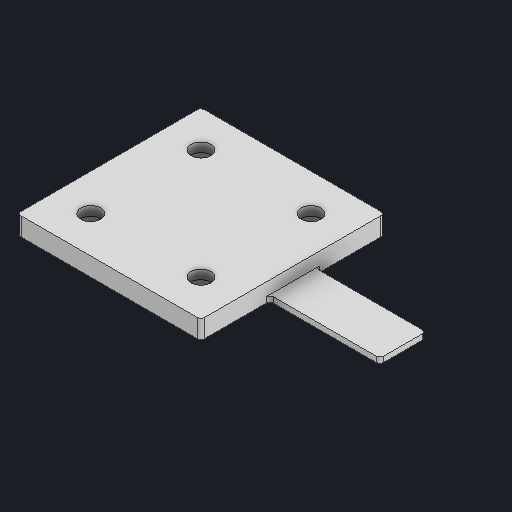
# Autodesk Inventor part: cradle_base
Saved by Autodesk Inventor 2025 (Build 290162010, 162A)
## iProperties
Created: 2024-06-21
Part Number: cradle_base
Material: Generic
Document SubType Name: Modeling
Designer: mihir
Density: 1 g/cm^3
Appearance: Default
Author: mihir
Autodesk Inventor part; units mm, degrees
ref_plane "YZ Plane" through (0, 0, 0) normal (1, 0, 0) x (0, 1, 0)
ref_plane "XZ Plane" through (0, 0, 0) normal (0, 1, 0) x (-1, 0, 0)
ref_plane "XY Plane" through (0, 0, 0) normal (0, 0, 1) x (1, 0, 0)
sketch "Sketch1" plane through (0, 0, 0) normal (0, 1, 0) x (-1, 0, 0)
  line L0 (100, 0) -> (0, 0)
  line L1 (0, 0) -> (0, -100)
  line L2 (0, -100) -> (100, -100)
  line L3 (100, -100) -> (100, 0)
  dimension "d0" = 100
  constraints: 8 end point, 2 parallel, 2 perpendicular, 1 coincident, 1 horizontal
  measures "d0" distance of L2.end L0.start
extrude "Extrusion1" add sketch "Sketch1" along normal blind 10
sketch "Sketch2" plane through (0, 10, 0) normal (0, 1, 0) x (1, 0, 0)
  line L0 (-20, 20) -> (-80, 20) construction
  line L1 (-80, 20) -> (-80, 80) construction
  line L2 (-80, 80) -> (-20, 80) construction
  line L3 (-20, 80) -> (-20, 20) construction
  line L4 (-100, 0) -> (0, 0) construction
  line L5 (0, 0) -> (0, 100) construction
  dimension "d3" = 60
  dimension "d4" = 20
  dimension "d5" = 20
  constraints: 8 end point, 2 perpendicular, 2 vertical, 1 horizontal
  measures "d3" distance of L2.end L0.start
  measures "d4" distance from line of L4 L0.start
  measures "d5" distance from line of L5 L0.start
hole "Hole1" at (-20, 10, -20) at (-80, 10, -20) at (-20, 10, -80) at (-80, 10, -80) direction (0, -1, 0) diameter 6.3 depth 7.5 tip angle 118
sketch "Sketch3" plane through (0, 10, 0) normal (0, 1, 0) x (1, 0, 0)
  circle A0 centre (-80, 20) radius 3.15 projected
  circle A1 centre (-20, 20) radius 3.15 projected
  circle A2 centre (-80, 80) radius 3.15 projected
  circle A3 centre (-20, 80) radius 3.15 projected
  point P0 (0, 0)
  constraints: 4 coincident
hole "Hole2" at (-80, 10, -20) at (-20, 10, -20) at (-80, 10, -80) at (-20, 10, -80) direction (0, -1, 0) diameter 10.8 depth 5 tip angle 118
fillet "Fillet1" radius 2 4 edges at (-100, 5, 0) (0, 5, 0) (0, 5, -100) (-100, 5, -100)
sketch "Sketch4" plane through (0, 0, 0) normal (0, -1, 0) x (1, 0, 0)
  line L0 (60, -37.5) -> (0, -37.5)
  line L1 (0, -37.5) -> (0, -62.5)
  line L2 (0, -62.5) -> (60, -62.5)
  line L3 (60, -62.5) -> (60, -37.5)
  line L4 (0, -2) -> (0, -98) projected
  line L5 (60, -50) -> (0, -50) construction
  line L6 (-98, 0) -> (-2, 0) construction
  point P0 (0, 0)
  dimension "d21" = 25
  dimension "d22" = 60
  dimension "d23" = 50
  constraints: 10 end point, 2 midpoint, 2 parallel, 2 perpendicular, 1 collinear, 1 horizontal
  measures "d21" distance of L2.end L0.start
  measures "d22" distance of L1.end L2.end
  measures "d23" distance between parallel lines of L6 L5
extrude "Extrusion2" add sketch "Sketch4" against normal blind 3
fillet "Fillet2" radius 2 4 edges at (0, 1.5, -37.5) (60, 1.5, -37.5) (60, 1.5, -62.5) (0, 1.5, -62.5)
equation "\"d0\" = base_width"
equation "\"d1\" = base_thickness"
equation "\"d3\" = rod_dist"
equation "\"d4\" = 0.5 * base_width - 0.5 * rod_dist"
equation "\"d5\" = 0.5 * base_width - 0.5 * rod_dist"
equation "\"d6\" = rod_tolerance + rod_diameter"
equation "\"d11\" = 0.75 * base_thickness"
equation "\"d13\" = rod_tolerance + post_diameter"
equation "\"d18\" = 0.5 * base_thickness"
equation "\"d21\" = flange_width"
equation "\"d22\" = flange_length"
equation "\"d23\" = 0.5 * base_width"
equation "\"base_width\" = 100"
equation "\"base_thickness\" = 10"
equation "\"rod_diameter\" = 6"
equation "\"rod_tolerance\" = 0.3"
equation "\"flange_length\" = 60"
equation "\"flange_width\" = 25"
equation "\"post_diameter\" = 10.5"
equation "\"rod_dist\" = 60"
body "Solid1"
